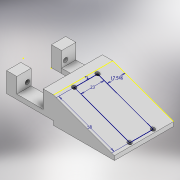
# Autodesk Inventor part: raspberry_holder
Saved by Autodesk Inventor 2021 (Build 250183000, 183)
## iProperties
Created: 2020-07-28
Part Number: raspberry_holder
Material: Generic
Document SubType Name: Modeling
Designer: Mazur
Density: 1 g/cm^3
Appearance: Default
Author: Mazur
Autodesk Inventor part; units mm, degrees
ref_plane "YZ Plane" through (0, 0, 0) normal (1, 0, 0) x (0, 1, 0)
ref_plane "XZ Plane" through (0, 0, 0) normal (0, 1, 0) x (-1, 0, 0)
ref_plane "XY Plane" through (0, 0, 0) normal (0, 0, 1) x (1, 0, 0)
sketch "Sketch1" plane through (0, 0, 0) normal (1, 0, 0) x (0, 1, 0)
  circle A0 centre (9.9082, -6.3418) radius 2.15
  circle A1 centre (9.9082, -6.3418) radius 2.15
  circle A2 centre (9.9082, -43.8418) radius 2.15
  circle A3 centre (9.9082, -43.8418) radius 2.15
  line L0 (19.9082, 0) -> (19.9082, -50.0918)
  line L1 (19.9082, -50.0918) -> (-0.0918, -50.0918)
  line L2 (-0.0918, -50.0918) -> (-0.0918, 0)
  line L3 (-0.0918, 0) -> (19.9082, 0)
  line L4 (19.9082, 0) -> (-0.0918, 0)
  line L5 (-0.0918, 0) -> (-0.0918, -10)
  line L6 (-0.0918, -10) -> (19.9082, -10)
  line L7 (19.9082, -10) -> (19.9082, 0)
  line L8 (19.9082, -50.0918) -> (-0.0918, -50.0918)
  line L9 (-0.0918, -50.0918) -> (-0.0918, -40.0918)
  line L10 (-0.0918, -40.0918) -> (19.9082, -40.0918)
  line L11 (19.9082, -40.0918) -> (19.9082, -50.0918)
  point P0 (0, 0)
  point P1 (19.9082, -50.0918)
  dimension "d0" = 10
  dimension "d1" = 10
  constraints: 24 end point, 6 parallel, 4 centre point, 3 perpendicular, 2 coincident, 2 horizontal, 2 point on line
  measures "d0" distance of L5.end L4.end
  measures "d1" distance of L8.end L9.end
extrude "Extrusion1" add sketch "Sketch1" along normal blind 10 contours L0 L6 L2 L3 | L0 L1 L2 L10
sketch "Sketch2" plane through (10, 0, 0) normal (1, 0, 0) x (0, 0, -1)
  line L0 (10, -0.0918) -> (10, 19.9082) projected
  line L1 (0, 19.9082) -> (0, -0.0918) projected
  line L2 (10, -0.0918) -> (0, -0.0918)
  line L3 (0, -0.0918) -> (0, 4.9082)
  line L4 (0, 4.9082) -> (10, 4.9082)
  line L5 (10, 4.9082) -> (10, -0.0918)
  line L6 (50.0697, -0.0918) -> (40.0697, -0.0918)
  line L7 (40.0697, -0.0918) -> (40.0697, 4.9082)
  line L8 (40.0697, 4.9082) -> (50.0697, 4.9082)
  line L9 (50.0697, 4.9082) -> (50.0697, -0.0918)
  point P0 (0, 0)
  dimension "d4" = 5
  dimension "d5" = 10
  dimension "d6" = 5
  constraints: 16 end point, 4 parallel, 2 horizontal, 2 perpendicular, 2 point on line
  measures "d4" distance of L2.end L3.end
  measures "d5" distance of L7.end L8.end
  measures "d6" distance of L6.end L7.end
extrude "Extrusion2" add sketch "Sketch2" along normal blind 26
thicken "Thicken1" operation add thickness 4 both sides no extend neighbours yes toward (0, 0, 1) faces at (3.3333, 8.2416, 0)
sketch "Sketch3" plane through (10, -0.0918, -40.0697) normal (0, 0, 1) x (1, 0, 0)
  point P0 (-10, 0.0918)
thicken "Thicken2" operation add thickness 4 both sides no extend neighbours yes toward (0, 0, -1) faces at (18.6667, 1.5749, -50.0697)
thicken "Thicken3" operation add thickness 4 both sides no extend neighbours yes toward (0, 0, -1) faces at (3.3333, 8.2416, -50.0918)
thicken "Thicken4" operation add thickness 0.4 both sides no extend neighbours yes toward (0, 1, 0) faces at (27.3333, -0.0918, -44.7437)
thicken "Thicken5" operation add thickness 0.4 both sides no extend neighbours yes toward (0, 1, 0) faces at (24, -0.0918, -0.6667)
sketch "Sketch4" plane through (36, 0, 0) normal (1, 0, 0) x (0, 0, -1)
  line L0 (-4, 4.9082) -> (-4, 0.3082) projected
  line L1 (54.0918, 0.3082) -> (54.0918, 19.9082) projected
  line L2 (-4, 0.3082) -> (54.0918, 0.3082)
  line L3 (54.0918, 0.3082) -> (54.0918, 10.3082)
  line L4 (54.0918, 10.3082) -> (-4, 10.3082)
  line L5 (-4, 10.3082) -> (-4, 0.3082)
  point P0 (0, 0)
  dimension "d19" = 10
  constraints: 8 end point, 2 parallel, 1 horizontal, 1 perpendicular, 1 point on line
  measures "d19" distance of L3.end L2.end
extrude "Extrusion3" add sketch "Sketch4" along normal blind 70
thicken "Thicken6" operation add thickness 12 both sides no extend neighbours yes toward (0, 1, 0) faces at (59.3333, 10.3082, -34.7278)
sketch "Sketch5" plane through (0, 0.3082, -54.0918) normal (0, -1, 0) x (1, 0, 0)
  line L0 (106, 58.0918) -> (106, 0) projected
  line L1 (0, 58.0918) -> (106, 58.0918) projected
  line L2 (106, 0) -> (46, 0)
  line L3 (46, 0) -> (46, 58.0918)
  line L4 (46, 58.0918) -> (106, 58.0918)
  line L5 (106, 58.0918) -> (106, 0)
  point P0 (0, 54.0918)
  dimension "d24" = 60
  constraints: 8 end point, 2 parallel, 1 horizontal, 1 perpendicular, 1 point on line
  measures "d24" distance of L3.end L4.end
extrude "Extrusion4" add sketch "Sketch5" along normal blind 4
chamfer "Chamfer2" distance 60 angle 20 1 edges at (106, 22.3082, -25.0459) measured on face at (105.5, 22.3082, -25.0459)
sketch "Sketch7" plane through (106, 0.47, 4) normal (0.3420201, 0.9396926, 0) x (0.9396926, -0.3420201, 0)
  line L0 (-60.8507, 17.5458) -> (-2.8507, 17.5458)
  line L1 (-2.8507, 17.5458) -> (-2.8507, 40.5458)
  line L2 (-2.8507, 40.5458) -> (-60.8507, 40.5458)
  line L3 (-60.8507, 40.5458) -> (-60.8507, 17.5458)
  line L4 (-63.8507, 58.0918) -> (-63.8507, 0) projected
  line L5 (0, 58.0918) -> (-63.8507, 58.0918) projected
  point P0 (-99.4467, 4)
  dimension "d33" = 23
  dimension "d34" = 58
  dimension "d35" = 3
  dimension "d36" = 17.546
  constraints: 8 end point, 2 parallel, 1 horizontal, 1 perpendicular
  measures "d33" distance of L2.end L0.start
  measures "d34" distance of L0.start L0.end
  measures "d35" distance between parallel lines of L4 L3
  measures "d36" distance between parallel lines of L5 L2
hole "Hole1" at (48.8191, 21.2822, -13.5458) at (48.8191, 21.2822, -36.5458) at (103.3212, 1.445, -36.5458) at (103.3212, 1.445, -13.5458) direction (-0.3420201, -0.9396926, 0) diameter 4 end through all
body "Solid1"
